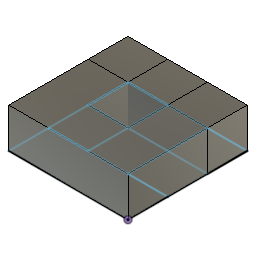
BooleanIntersectMultiOverlap (Autodesk Fusion 360 design; units mm, degrees)
Autodesk Fusion 360 part; units mm, degrees
sketch "Sketch1" plane through (0, 0, 0) normal (0, 0, 1) x (1, 0, 0)
  line L0 (0, 0) -> (-30, 0)
  line L1 (-30, 0) -> (-30, 10)
  line L2 (-30, 10) -> (0, 10)
  line L3 (0, 10) -> (0, 0)
  line L4 (-30, 10) -> (-20, 10)
  line L5 (-20, 10) -> (-20, 30)
  line L6 (-20, 30) -> (-30, 30)
  line L7 (-30, 30) -> (-30, 10)
  line L8 (0, 10) -> (-10, 10)
  line L9 (-10, 10) -> (-10, 30)
  line L10 (-10, 30) -> (0, 30)
  line L11 (0, 30) -> (0, 10)
  line L12 (-30, 30) -> (0, 30)
  line L13 (0, 30) -> (0, 20)
  line L14 (0, 20) -> (-30, 20)
  line L15 (-30, 20) -> (-30, 30)
  constraint horizontal L0
  constraint vertical L1
  constraint horizontal L2
  constraint vertical L3
  constraint coincident L0.start L3.end
  constraint horizontal L4
  constraint vertical L5
  constraint horizontal L6
  constraint vertical L7
  constraint horizontal L8
  constraint vertical L9
  constraint horizontal L10
  constraint vertical L11
  constraint horizontal L12
  constraint vertical L13
  constraint horizontal L14
  constraint vertical L15
  constraint midpoint L11 L13.end
extrude "Extrude1" add sketch "Sketch1" along normal blind 10 contours L0 L1 L2 L3 L4 L8 | L2 L8 L9 L11 L14 | L2 L4 L5 L7 L14 | L9 L10 L11 L12 L13 L14 | L5 L6 L7 L12 L14 L15 makes body 1
extrude "Extrude1'" add sketch "Sketch1" along normal blind 10 separate body contours L9 L10 L11 L12 L13 L14 | L5 L6 L7 L12 L14 L15 | L5 L9 L12 L14 makes body 2 in component "Tool"
component "Tool" placed x (1, 0, 0) y (0, 1, 0) z (0, 0, 1) at (0, 0, 0)
